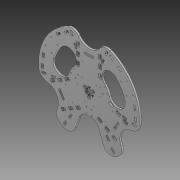
# Autodesk Inventor part: Корпус_В2_Основание
Saved by Autodesk Inventor 2022 (Build 260153000, 153)
## iProperties
Created: 2025-01-10
Part Number: Корпус_В2_Основание
Material: Типовые
Document SubType Name: Modeling
Designer: Ivan
Density: 1 g/cm^3
Appearance: Гладкий — нейтральный серый
Mass: 388.916 g
Surface Area: 1549.84 cm^2
Volume: 388.916 cm^3
Author: Ivan
Title: Корпус_В2_Основание
Autodesk Inventor part; units mm, degrees
ref_plane "YZ Plane" through (0, 0, 0) normal (1, 0, 0) x (0, 1, 0)
ref_plane "XZ Plane" through (0, 0, 0) normal (0, 1, 0) x (-1, 0, 0)
ref_plane "РабПлоскость1" through (38, -105, -570.6896) normal (0, 0, -1) x (-1, 0, 0)
sketch "Эскиз1" plane through (38, -105, -570.6896) normal (0, 0, -1) x (-1, 0, 0)
  line L0 (38, 105) -> (38, -150.1213) construction
  circle A0 centre (38, -75) radius 180
  ellipse E0 centre (38, 104.9513) end of major axis (84.5, 104.9513) minor radius 46.5 projected
  circle A1 centre (38, 104.9513) radius 46.5
  circle A2 centre (-117.8424, -164.9757) radius 46.5
  circle A3 centre (193.8424, -164.9757) radius 46.5
  point P0 (84.1166, 98.9921)
  point P1 (-8.1166, 98.9921)
  point P2 (165.6233, -201.9342)
  point P3 (211.7399, -122.0579)
  point P4 (84.1166, 98.9921)
  point P5 (84.5, 104.9513)
  point P6 (-8.1166, 98.9921)
  point P7 (-8.5, 104.9513)
  point P8 (-135.7399, -122.0579)
  point P9 (-89.6233, -201.9342)
  dimension "d0" = 180
  dimension "d6" = 360
  constraints: 3 centre point, 2 end point, 1 coincident, 1 point on line, 1 vertical, 12 other
  measures "d0" distance of point (38, -75) L0.start
extrude "Выдавливание1" add sketch "Эскиз1" along normal blind 6 contours A0 A3 A2 E0
fillet "Сопряжение1" radius 30 6 edges at (-173.7399, -227.0579, -573.6896) (-127.6233, -306.9342, -573.6896) (127.6233, -306.9342, -573.6896) (173.7399, -227.0579, -573.6896) (-46.1166, -6.0079, -573.6896) (46.1166, -6.0079, -573.6896)
sketch "Эскиз2" plane through (38, -105, -570.6896) normal (0, 0, 1) x (1, 0, 0)
  arc A0 (37.3316, 88.4783) -> (0.1581, 78.3768) centre (24.7763, 61.2319) ccw construction
  arc A1 (-76.1581, 78.3768) -> (0.1581, 78.3768) centre (-38, 104.9513) ccw construction
  arc A2 (-76.1581, 78.3768) -> (-113.3316, 88.4783) centre (-100.7763, 61.2319) ccw construction
  arc A3 (-113.3316, 88.4783) -> (-217.2421, -91.5001) centre (-38, -75) ccw construction
  arc A4 (-217.2421, -91.5001) -> (-189.9073, -118.6425) centre (-187.3685, -88.7501) ccw construction
  arc A5 (-151.7491, -184.7343) -> (-189.9073, -118.6425) centre (-193.8424, -164.9757) ccw construction
  arc A6 (-151.7491, -184.7343) -> (-141.9106, -221.9782) centre (-124.5921, -197.4818) ccw construction
  arc A7 (-141.9106, -221.9782) -> (65.9106, -221.9782) centre (-38, -75) ccw construction
  arc A8 (65.9106, -221.9782) -> (75.7491, -184.7343) centre (48.5921, -197.4818) ccw construction
  arc A9 (113.9073, -118.6425) -> (75.7491, -184.7343) centre (117.8424, -164.9757) ccw construction
  arc A10 (113.9073, -118.6425) -> (141.2421, -91.5001) centre (111.3685, -88.7501) ccw construction
  arc A11 (141.2421, -91.5001) -> (37.3316, 88.4783) centre (-38, -75) ccw construction
  circle A12 centre (-38, -75) radius 133
  circle A13 centre (-38, -75) radius 75
  line L0 (-38, -75) -> (28.5, 40.1814)
  line L1 (-38, -75) -> (95, -75)
  line L2 (-38, -75) -> (-38, -366.3532) construction
  line L3 (-38, -75) -> (208.094, 67.0824) construction
  circle A14 centre (-38, -75) radius 104 construction
  line L4 (-0.5, -10.0481) -> (28.5, 40.1814) construction
  point P0 (-38, 105)
  point P1 (37, -75)
  point P2 (-0.5, -10.0481)
  point P3 (14, 15.0666)
  dimension "d9" = 150
  dimension "d52" = 208
  dimension "d8" = 58
  dimension "d10" = 60
  dimension "d11" = 120
  constraints: 10 end point, 3 coincident, 2 point on circle, 1 centre point, 1 midpoint, 1 point on line, 1 vertical, 7 other
  measures "d10" angle of L1 L0
  measures "d11" angle of L2 L3
extrude "Выдавливание2" cut sketch "Эскиз2" against normal through all contours L1 A13 L0 A12 picked at (61.1819, -19.8946)
fillet "Сопряжение2" radius 29 4 edges at (37.5, -115.0481, -573.6896) (66.5, -64.8186, -573.6896) (75, -180, -573.6896) (133, -180, -573.6896)
mirror "Зеркальное отражение1" about plane through (0, 0, 0) normal (1, 0, 0) of "Сопряжение2", "Выдавливание2"
sketch "Эскиз3" plane through (38, -105, -570.6896) normal (0, 0, 1) x (1, 0, 0)
  circle A0 centre (-38, -75) radius 75 projected
  circle A1 centre (-38, -75) radius 133 construction
  line L0 (-38, -75) -> (25.1637, -248.5408)
  line L1 (-38, -75) -> (-101.1637, -248.5408)
  line L2 (-38, -75) -> (-38, -284.9375) construction
  circle A2 centre (-38, -75) radius 184.6782
  point P0 (-38, 105)
  point P1 (-12.3485, -145.4769)
  point P2 (-63.6515, -145.4769)
  dimension "d15" = 40
  constraints: 6 end point, 2 point on circle, 1 centre point, 1 coincident, 1 vertical, 1 other
  measures "d15" angle of L0 L1
extrude "Выдавливание3" cut sketch "Эскиз3" against normal through all contours A0 L0 A2 L1 picked at (-36.2561, -222.9049)
fillet "Сопряжение3" radius 30 4 edges at (-25.6515, -250.4769, -573.6896) (-61.5636, -349.1447, -573.6896) (25.6515, -250.4769, -573.6896) (61.5636, -349.1447, -573.6896)
sketch "Эскиз4" plane through (38, -105, -570.6896) normal (0, 0, 1) x (1, 0, 0)
  arc A0 (12.2665, -213.106) -> (56.1487, -228.4145) centre (40.4573, -202.8454) ccw construction
  arc A1 (65.9106, -221.9782) -> (75.7491, -184.7343) centre (48.5921, -197.4818) ccw construction
  arc A2 (113.9073, -118.6425) -> (75.7491, -184.7343) centre (117.8424, -164.9757) ccw construction
  arc A3 (113.9073, -118.6425) -> (141.2421, -91.5001) centre (111.3685, -88.7501) ccw construction
  arc A4 (141.2421, -91.5001) -> (37.3316, 88.4783) centre (-38, -75) ccw construction
  arc A5 (37.3316, 88.4783) -> (0.1581, 78.3768) centre (24.7763, 61.2319) ccw construction
  arc A6 (-76.1581, 78.3768) -> (0.1581, 78.3768) centre (-38, 104.9513) ccw construction
  arc A7 (-76.1581, 78.3768) -> (-113.3316, 88.4783) centre (-100.7763, 61.2319) ccw construction
  arc A8 (-113.3316, 88.4783) -> (-217.2421, -91.5001) centre (-38, -75) ccw construction
  arc A9 (-217.2421, -91.5001) -> (-189.9073, -118.6425) centre (-187.3685, -88.7501) ccw construction
  arc A10 (-151.7491, -184.7343) -> (-189.9073, -118.6425) centre (-193.8424, -164.9757) ccw construction
  arc A11 (-151.7491, -184.7343) -> (-141.9106, -221.9782) centre (-124.5921, -197.4818) ccw construction
  arc A12 (-132.1487, -228.4145) -> (-88.2665, -213.106) centre (-116.4573, -202.8454) ccw construction
  line L0 (-88.2665, -213.106) -> (-72.4151, -169.5547) construction
  arc A13 (-42.446, -149.8681) -> (-72.4151, -169.5547) centre (-44.2243, -179.8154) ccw construction
  arc A14 (-42.446, -149.8681) -> (-33.554, -149.8681) centre (-38, -75) ccw construction
  arc A15 (-3.5849, -169.5547) -> (-33.554, -149.8681) centre (-31.7757, -179.8154) ccw construction
  line L1 (-3.5849, -169.5547) -> (12.2665, -213.106) construction
  arc A16 (-133.9802, 17.0695) -> (-165.7247, -37.9135) centre (-38, -75) ccw construction
  arc A17 (-92.1242, -23.0811) -> (-110.0252, -54.0865) centre (-38, -75) ccw construction
  arc A18 (89.7247, -37.9135) -> (57.9802, 17.0695) centre (-38, -75) ccw construction
  arc A19 (34.0252, -54.0865) -> (16.1242, -23.0811) centre (-38, -75) ccw construction
  circle A20 centre (-38, -75) radius 20
  circle A21 centre (-38, -8.9997) radius 2 construction
  line L2 (-38, -8.9997) -> (-38, -75) construction
  line L3 (-38, -75) -> (8.5542, -48.1219) construction
  arc A22 (18.8589, -105.5181) -> (21.457, -107.0181) centre (19.1579, -108.0002) ccw construction
  line L4 (-38, -8.9997) -> (19.1579, -108.0002) construction
  circle A23 centre (-23.2776, -66.5) radius 5
  circle A24 centre (-38, -75) radius 17 construction
  line L5 (-28.1932, -65.5853) -> (-30.524, -66.931)
  line L6 (-24.9432, -71.2144) -> (-27.274, -72.5601)
  circle A25 centre (-38, -75) radius 11
  line L7 (-47.8068, -65.5853) -> (-45.476, -66.931)
  line L8 (-51.0568, -71.2144) -> (-48.726, -72.5601)
  circle A26 centre (-52.7224, -66.5) radius 5
  line L9 (-41.25, -88.2003) -> (-41.25, -85.5089)
  line L10 (-34.75, -88.2003) -> (-34.75, -85.5089)
  circle A27 centre (-38, -92) radius 5
  line L11 (-43, -59) -> (-33, -59)
  line L12 (-33, -59) -> (-33, -61)
  line L13 (-33, -61) -> (-43, -61)
  line L14 (-43, -61) -> (-43, -59)
  line L15 (-43, -59) -> (-33, -61) construction
  line L16 (-33, -59) -> (-43, -61) construction
  line L17 (-37, -61) -> (-37, -64.0455)
  line L18 (-39, -61) -> (-39, -64.0455)
  line L19 (-49.6244, -82.866) -> (-46.9868, -81.3433)
  line L20 (-50.6244, -81.134) -> (-47.9868, -79.6112)
  line L21 (-54.3564, -78.6699) -> (-52.6244, -77.6699)
  line L22 (-47.6244, -86.3301) -> (-49.3564, -87.3301)
  line L23 (-52.6244, -77.6699) -> (-47.6244, -86.3301)
  line L24 (-49.3564, -87.3301) -> (-54.3564, -78.6699)
  line L25 (-49.3564, -87.3301) -> (-52.6244, -77.6699) construction
  line L26 (-54.3564, -78.6699) -> (-47.6244, -86.3301) construction
  line L27 (-25.3756, -81.134) -> (-28.0132, -79.6112)
  line L28 (-26.3756, -82.866) -> (-29.0132, -81.3433)
  line L29 (-26.6436, -87.3301) -> (-28.3756, -86.3301)
  line L30 (-23.3756, -77.6699) -> (-21.6436, -78.6699)
  line L31 (-28.3756, -86.3301) -> (-23.3756, -77.6699)
  line L32 (-21.6436, -78.6699) -> (-26.6436, -87.3301)
  line L33 (-21.6436, -78.6699) -> (-28.3756, -86.3301) construction
  line L34 (-26.6436, -87.3301) -> (-23.3756, -77.6699) construction
  arc A28 (-165.7247, -37.9135) -> (-110.0252, -54.0865) centre (-137.8749, -46) ccw projected
  arc A29 (-92.1242, -23.0811) -> (-133.9802, 17.0695) centre (-113.0522, -3.0058) ccw projected
  arc A30 (57.9802, 17.0695) -> (16.1242, -23.0811) centre (37.0522, -3.0058) ccw projected
  arc A31 (34.0252, -54.0865) -> (89.7247, -37.9135) centre (61.8749, -46) ccw projected
  arc A32 (56.1487, -228.4145) -> (65.9106, -221.9782) centre (-38, -75) ccw projected
  arc A33 (-141.9106, -221.9782) -> (-132.1487, -228.4145) centre (-38, -75) ccw projected
  point P0 (-38, 105)
  point P1 (-38, -60)
  point P2 (-50.9904, -82.5)
  point P3 (-25.0096, -82.5)
  point P4 (-28.0132, -79.6112)
  point P5 (-45.476, -66.931)
  point P6 (-47.9868, -79.6112)
  point P7 (-46.9868, -81.3433)
  point P8 (-41.25, -85.5089)
  point P9 (-29.0132, -81.3433)
  dimension "d21" = 34
  dimension "d19" = 40
  dimension "d20" = 10
  dimension "d22" = 6.5
  dimension "d23" = 22
  dimension "d26" = 360
  dimension "d28" = 10
  dimension "d29" = 2
  dimension "d30" = 2
  dimension "d31" = 15
  dimension "d34" = 360
  constraints: 66 end point, 10 point on circle, 8 point on line, 6 midpoint, 5 centre point, 4 parallel, 3 coincident, 2 perpendicular, 2 vertical, 1 horizontal, 82 other
  measures "d19" diameter of A20
  measures "d20" diameter of A23
  measures "d22" distance between parallel lines of L5 L6
  measures "d23" diameter of A25
  measures "d28" distance of L12.end L13.end
  measures "d29" distance of L11.end L12.end
  measures "d30" distance between parallel lines of L18 L17
  measures "d31" distance of A16.centre point (-38, -60)
extrude "Выдавливание4" cut sketch "Эскиз4" against normal through all contours A23 A20 | A20 A23 | A27 A20 | A20 A27 | L6 A25 L5 A23 | A26 A20 | A20 A26 | A25 | L9 A25 L10 A27 | L7 A25 L8 A26 | A25 L18 L13 L17 | L27 L31 L28 A25 | L19 L23 L20 A25 | L13 L14 L11 L12 | L31 L30 L32 L29 | L23 L22 L24 L21
fillet "Сопряжение4" radius 1 24 edges at (9.9868, -184.6112, -573.6896) (8.9868, -186.3433, -573.6896) (10.726, -177.5601, -573.6896) (7.476, -171.931, -573.6896) (1, -169.0455, -573.6896) (-1, -169.0455, -573.6896) (-7.476, -171.931, -573.6896) (-10.726, -177.5601, -573.6896) (-8.9868, -186.3433, -573.6896) (-9.9868, -184.6112, -573.6896) (-3.25, -190.5089, -573.6896) (3.25, -190.5089, -573.6896) (11.6244, -187.866, -573.6896) (12.6244, -186.134, -573.6896) (-11.6244, -187.866, -573.6896) (-12.6244, -186.134, -573.6896) (1, -166, -573.6896) (-1, -166, -573.6896) (-9.8068, -170.5853, -573.6896) (-13.0568, -176.2144, -573.6896) (9.8068, -170.5853, -573.6896) (13.0568, -176.2144, -573.6896) (3.25, -193.2003, -573.6896) (-3.25, -193.2003, -573.6896)
sketch "Эскиз5" plane through (38, -105, -576.6896) normal (0, 0, -1) x (-1, 0, 0)
  arc A0 (217.2421, -91.5001) -> (113.3316, 88.4783) centre (38, -75) ccw construction
  arc A1 (217.2421, -91.5001) -> (113.3316, 88.4783) centre (38, -75) ccw construction
  arc A2 (36.1667, -64.1539) -> (31.0391, -66.4826) centre (38, -75) ccw construction
  arc A3 (88.2665, -213.106) -> (132.1487, -228.4145) centre (116.4573, -202.8454) ccw construction
  line L0 (38, -75) -> (116.4573, -202.8454) construction
  line L1 (124.3613, -221.4606) -> (98.2089, -178.8455)
  line L2 (98.2089, -178.8455) -> (103.3227, -175.7072)
  line L3 (103.3227, -175.7072) -> (129.4751, -218.3224)
  line L4 (129.4751, -218.3224) -> (124.3613, -221.4606)
  line L5 (124.3613, -221.4606) -> (103.3227, -175.7072) construction
  line L6 (98.2089, -178.8455) -> (129.4751, -218.3224) construction
  line L7 (106.0546, -191.63) -> (111.1685, -188.4918)
  line L8 (121.6294, -205.5378) -> (116.5156, -208.6761)
  line L9 (113.842, -198.5839) -> (116.3989, -197.0148) construction
  circle A4 centre (38, -75) radius 145 construction
  line L10 (38, -75) -> (215.7726, -98.4042) construction
  arc A5 (189.9073, -118.6425) -> (217.2421, -91.5001) centre (187.3685, -88.7501) ccw construction
  line L11 (38, -75) -> (106.6177, 90.6577) construction
  arc A6 (113.3316, 88.4783) -> (76.1581, 78.3768) centre (100.7763, 61.2319) ccw construction
  line L12 (38, -75) -> (193.8846, 15) construction
  arc A7 (217.2421, -91.5001) -> (113.3316, 88.4783) centre (38, -75) ccw construction
  line L13 (206.154, -100.1638) -> (156.5818, -93.6375)
  line L14 (156.5818, -93.6375) -> (157.365, -87.6888)
  line L15 (157.365, -87.6888) -> (206.9372, -94.2151)
  line L16 (206.9372, -94.2151) -> (206.154, -100.1638)
  line L17 (206.154, -100.1638) -> (157.365, -87.6888) construction
  line L18 (156.5818, -93.6375) -> (206.9372, -94.2151) construction
  line L19 (171.4535, -95.5954) -> (172.2366, -89.6467)
  line L20 (192.0655, -92.2572) -> (191.2824, -98.2059)
  line L21 (181.7595, -93.9263) -> (182.1511, -90.952) construction
  line L22 (81.1504, 37.0136) -> (100.2845, 83.2076)
  line L23 (100.2845, 83.2076) -> (105.8278, 80.9115)
  line L24 (105.8278, 80.9115) -> (86.6937, 34.7175)
  line L25 (86.6937, 34.7175) -> (81.1504, 37.0136)
  line L26 (81.1504, 37.0136) -> (105.8278, 80.9115) construction
  line L27 (100.2845, 83.2076) -> (86.6937, 34.7175) construction
  line L28 (94.5443, 69.3494) -> (100.0876, 67.0533)
  line L29 (92.4339, 48.5757) -> (86.8906, 50.8718)
  line L30 (93.4891, 58.9625) -> (96.2607, 57.8145) construction
  line L31 (203.1818, -35.453) -> (207.5396, -85.2627)
  line L32 (207.5396, -85.2627) -> (201.5624, -85.7856)
  line L33 (201.5624, -85.7856) -> (197.2046, -35.9759)
  line L34 (197.2046, -35.9759) -> (203.1818, -35.453)
  line L35 (203.1818, -35.453) -> (201.5624, -85.7856) construction
  line L36 (207.5396, -85.2627) -> (197.2046, -35.9759) construction
  line L37 (206.2323, -70.3198) -> (200.2551, -70.8427)
  line L38 (204.4892, -50.3959) -> (198.512, -50.9188)
  line L39 (202.3721, -60.6193) -> (199.3835, -60.8808) construction
  circle A8 centre (38, -75) radius 165 construction
  line L40 (202.3721, -60.6193) -> (204.551, -85.5242) construction
  line L41 (38, -75) -> (38, 24.0008) construction
  line L42 (154.8396, 48.2781) -> (113.882, 76.957)
  line L43 (113.882, 76.957) -> (110.4406, 72.042)
  line L44 (110.4406, 72.042) -> (151.3982, 43.3632)
  line L45 (151.3982, 43.3632) -> (154.8396, 48.2781)
  line L46 (154.8396, 48.2781) -> (110.4406, 72.042) construction
  line L47 (113.882, 76.957) -> (151.3982, 43.3632) construction
  line L48 (126.1693, 68.3533) -> (122.7279, 63.4384)
  line L49 (142.5524, 56.8818) -> (139.1109, 51.9669)
  line L50 (132.6401, 60.1601) -> (130.9194, 57.7026) construction
  line L51 (132.6401, 60.1601) -> (112.1613, 74.4995) construction
  point P0 (38, 105)
  point P1 (132.127, -206.5631)
  point P2 (156.9734, -90.6631)
  point P3 (93.4891, 58.9625)
  point P4 (103.0562, 82.0595)
  dimension "d60" = 330
  dimension "d39" = 6
  dimension "d40" = 50
  dimension "d41" = 15
  dimension "d42" = 290
  dimension "d45" = 75
  dimension "d46" = 6
  dimension "d47" = 50
  dimension "d48" = 15
  dimension "d49" = 6
  dimension "d50" = 50
  dimension "d51" = 15
  dimension "d58" = 15
  dimension "d59" = 15
  dimension "d61" = 85
  constraints: 104 end point, 25 point on line, 20 midpoint, 13 perpendicular, 12 symmetric about line, 8 parallel, 7 point on circle, 2 coincident, 2 equal length, 1 centre point, 1 vertical, 8 other
  measures "d39" distance of L3.end L1.start
  measures "d40" distance of L2.end L3.end
  measures "d41" distance between parallel lines of L4 L8
  measures "d42" diameter of A4
  measures "d45" angle of L11 L10
  measures "d46" distance of L15.end L16.end
  measures "d47" distance of L14.end L15.end
  measures "d48" distance between parallel lines of L16 L20
  measures "d49" distance of L24.end L25.end
  measures "d50" distance of L23.end L24.end
  measures "d51" distance between parallel lines of L25 L29
  measures "d58" distance between parallel lines of L34 L38
  measures "d59" distance between parallel lines of L32 L37
  measures "d61" angle of L39 L41
extrude "Выдавливание5" cut sketch "Эскиз5" against normal through all contours L1 L8 L3 L4 | L1 L2 L3 L7 | L13 L20 L15 L16 | L13 L14 L15 L19 | L22 L29 L24 L25 | L22 L23 L24 L28 | L31 L38 L33 L34 | L31 L32 L33 L37 | L45 L44 L49 L42 | L48 L44 L43 L42
mirror "Зеркальное отражение2" about plane through (0, 0, 0) normal (1, 0, 0) of "Выдавливание5"
sketch "Эскиз6" plane through (38, -105, -570.6896) normal (0, 0, 1) x (1, 0, 0)
  line L0 (100.9134, -104.3949) -> (87.923, -96.8949) projected
  line L1 (99.4134, -106.993) -> (100.9134, -104.3949) projected
  line L2 (86.423, -99.493) -> (87.923, -96.8949) projected
  line L3 (83.423, -104.6891) -> (84.923, -102.091) projected
  line L4 (84.923, -102.091) -> (86.423, -99.493) projected
  line L5 (97.9134, -109.591) -> (99.4134, -106.993) projected
  line L6 (96.4134, -112.1891) -> (97.9134, -109.591) projected
  line L7 (96.4134, -112.1891) -> (83.423, -104.6891) projected
  line L8 (73.4327, -91.993) -> (74.9327, -89.3949) projected
  line L9 (74.9327, -89.3949) -> (61.9423, -81.8949) projected
  line L10 (71.9327, -94.591) -> (73.4327, -91.993) projected
  line L11 (70.4327, -97.1891) -> (71.9327, -94.591) projected
  line L12 (70.4327, -97.1891) -> (57.4423, -89.6891) projected
  line L13 (57.4423, -89.6891) -> (58.9423, -87.091) projected
  line L14 (58.9423, -87.091) -> (60.4423, -84.493) projected
  line L15 (60.4423, -84.493) -> (61.9423, -81.8949) projected
  line L16 (49.7628, -142.9904) -> (64.7628, -117.0096) projected
  line L17 (64.7628, -117.0096) -> (69.9589, -120.0096) projected
  line L18 (54.9589, -145.9904) -> (69.9589, -120.0096) projected
  line L19 (49.7628, -142.9904) -> (54.9589, -145.9904) projected
  line L20 (48.423, -165.3109) -> (61.4134, -172.8109) projected
  line L21 (61.4134, -172.8109) -> (59.9134, -175.409) projected
  line L22 (46.923, -167.909) -> (59.9134, -175.409) projected
  line L23 (48.423, -165.3109) -> (46.923, -167.909) projected
  line L24 (46.923, -167.909) -> (59.9134, -175.409) projected
  line L25 (59.9134, -175.409) -> (58.4134, -178.007) projected
  line L26 (45.423, -170.507) -> (58.4134, -178.007) projected
  line L27 (46.923, -167.909) -> (45.423, -170.507) projected
  line L28 (45.423, -170.507) -> (58.4134, -178.007) projected
  line L29 (58.4134, -178.007) -> (56.9134, -180.6051) projected
  line L30 (43.923, -173.1051) -> (56.9134, -180.6051) projected
  line L31 (45.423, -170.507) -> (43.923, -173.1051) projected
  line L32 (22.4423, -150.3109) -> (35.4327, -157.8109) projected
  line L33 (35.4327, -157.8109) -> (33.9327, -160.409) projected
  line L34 (20.9423, -152.909) -> (33.9327, -160.409) projected
  line L35 (22.4423, -150.3109) -> (20.9423, -152.909) projected
  line L36 (20.9423, -152.909) -> (33.9327, -160.409) projected
  line L37 (33.9327, -160.409) -> (32.4327, -163.007) projected
  line L38 (19.4423, -155.507) -> (32.4327, -163.007) projected
  line L39 (20.9423, -152.909) -> (19.4423, -155.507) projected
  line L40 (19.4423, -155.507) -> (32.4327, -163.007) projected
  line L41 (32.4327, -163.007) -> (30.9327, -165.6051) projected
  line L42 (17.9423, -158.1051) -> (30.9327, -165.6051) projected
  line L43 (19.4423, -155.507) -> (17.9423, -158.1051) projected
  line L44 (99.4134, -106.993) -> (86.423, -99.493) projected
  line L45 (86.423, -99.493) -> (87.923, -96.8949) projected
  line L46 (100.9134, -104.3949) -> (87.923, -96.8949) projected
  line L47 (99.4134, -106.993) -> (100.9134, -104.3949) projected
  line L48 (97.9134, -109.591) -> (84.923, -102.091) projected
  line L49 (84.923, -102.091) -> (86.423, -99.493) projected
  line L50 (99.4134, -106.993) -> (86.423, -99.493) projected
  line L51 (97.9134, -109.591) -> (99.4134, -106.993) projected
  line L52 (96.4134, -112.1891) -> (83.423, -104.6891) projected
  line L53 (83.423, -104.6891) -> (84.923, -102.091) projected
  line L54 (97.9134, -109.591) -> (84.923, -102.091) projected
  line L55 (96.4134, -112.1891) -> (97.9134, -109.591) projected
  line L56 (47.4519, -76.993) -> (34.4615, -69.493) projected
  line L57 (34.4615, -69.493) -> (35.9615, -66.8949) projected
  line L58 (48.9519, -74.3949) -> (35.9615, -66.8949) projected
  line L59 (47.4519, -76.993) -> (48.9519, -74.3949) projected
  line L60 (45.9519, -79.591) -> (32.9615, -72.091) projected
  line L61 (32.9615, -72.091) -> (34.4615, -69.493) projected
  line L62 (47.4519, -76.993) -> (34.4615, -69.493) projected
  line L63 (45.9519, -79.591) -> (47.4519, -76.993) projected
  line L64 (44.4519, -82.1891) -> (31.4615, -74.6891) projected
  line L65 (31.4615, -74.6891) -> (32.9615, -72.091) projected
  line L66 (45.9519, -79.591) -> (32.9615, -72.091) projected
  line L67 (44.4519, -82.1891) -> (45.9519, -79.591) projected
  line L68 (73.4327, -91.993) -> (60.4423, -84.493) projected
  line L69 (60.4423, -84.493) -> (61.9423, -81.8949) projected
  line L70 (74.9327, -89.3949) -> (61.9423, -81.8949) projected
  line L71 (73.4327, -91.993) -> (74.9327, -89.3949) projected
  line L72 (70.4327, -97.1891) -> (57.4423, -89.6891) projected
  line L73 (57.4423, -89.6891) -> (58.9423, -87.091) projected
  line L74 (71.9327, -94.591) -> (58.9423, -87.091) projected
  line L75 (70.4327, -97.1891) -> (71.9327, -94.591) projected
  line L76 (71.9327, -94.591) -> (58.9423, -87.091) projected
  line L77 (58.9423, -87.091) -> (60.4423, -84.493) projected
  line L78 (73.4327, -91.993) -> (60.4423, -84.493) projected
  line L79 (71.9327, -94.591) -> (73.4327, -91.993) projected
  line L80 (-3.5385, -135.3109) -> (9.4519, -142.8109) projected
  line L81 (9.4519, -142.8109) -> (7.9519, -145.409) projected
  line L82 (-5.0385, -137.909) -> (7.9519, -145.409) projected
  line L83 (-3.5385, -135.3109) -> (-5.0385, -137.909) projected
  line L84 (-5.0385, -137.909) -> (7.9519, -145.409) projected
  line L85 (7.9519, -145.409) -> (6.4519, -148.007) projected
  line L86 (-6.5385, -140.507) -> (6.4519, -148.007) projected
  line L87 (-5.0385, -137.909) -> (-6.5385, -140.507) projected
  line L88 (-6.5385, -140.507) -> (6.4519, -148.007) projected
  line L89 (6.4519, -148.007) -> (4.9519, -150.6051) projected
  line L90 (-8.0385, -143.1051) -> (4.9519, -150.6051) projected
  line L91 (-6.5385, -140.507) -> (-8.0385, -143.1051) projected
  point P0 (-38, 105)
  constraints: 1 other
extrude "Выдавливание6" cut sketch "Эскиз6" against normal through all
pattern_circular "Круговой массив1" count 3 over 360 about axis through (0, -180, -570.6896) along (0, 0, -1) of "Выдавливание6"
sketch "Эскиз7" plane through (38, -105, -570.6896) normal (0, 0, 1) x (1, 0, 0)
  arc A0 (-113.3316, 88.4783) -> (-217.2421, -91.5001) centre (-38, -75) ccw projected
  line L0 (162, -225) -> (-238, -225)
  line L1 (-238, -225) -> (-238, 75)
  line L2 (-238, 75) -> (162, 75)
  line L3 (162, 75) -> (162, -225)
  line L4 (162, -225) -> (-238, 75) construction
  line L5 (-238, -225) -> (162, 75) construction
  line L6 (220.7514, -288.1285) -> (-335.7827, -288.1285)
  line L7 (-335.7827, -288.1285) -> (-335.7827, 148.337)
  line L8 (-335.7827, 148.337) -> (220.7514, 148.337)
  line L9 (220.7514, 148.337) -> (220.7514, -288.1285)
  point P0 (-38, 105)
  dimension "d64" = 300
  dimension "d65" = 400
  constraints: 20 end point, 4 parallel, 2 horizontal, 2 midpoint, 2 perpendicular
  measures "d64" distance of L0.end L1.end
  measures "d65" distance of L0.start L0.end
extrude "Выдавливание7" [suppressed]
sketch "Эскиз8" plane through (38, -105, -570.6896) normal (0, 0, 1) x (1, 0, 0)
  circle A0 centre (-13, -42.5) radius 3 construction
  circle A1 centre (-13, 7.5) radius 3 construction
  circle A2 centre (-63, -42.5) radius 3 construction
  circle A3 centre (-63, 7.5) radius 3 construction
  point P0 (-38, 105)
  constraints: 4 coincident
hole "Отверстие1" at (25, -147.5, -570.6896) at (25, -97.5, -570.6896) at (-25, -147.5, -570.6896) at (-25, -97.5, -570.6896) direction (0, 0, -1) diameter 1.5 end through all
pattern_circular "Круговой массив2" count 3 over 360 about axis through (0, -180, -570.6896) along (0, 0, -1) of "Отверстие1"
sketch "Эскиз9" plane through (38, -105, -570.6896) normal (0, 0, 1) x (1, 0, 0)
  arc A0 (56.1487, -228.4145) -> (65.9106, -221.9782) centre (-38, -75) ccw construction
  line L0 (-38, -75) -> (-38, -194.1828) construction
  line L1 (-29, -144) -> (-47, -144) construction
  line L2 (-47, -144) -> (-47, -126) construction
  line L3 (-47, -126) -> (-29, -126) construction
  line L4 (-29, -126) -> (-29, -144) construction
  line L5 (-29, -144) -> (-47, -126) construction
  line L6 (-47, -144) -> (-29, -126) construction
  circle A1 centre (-38, -75) radius 60 construction
  point P0 (-38, 105)
  point P1 (-217.2421, -91.5001)
  point P2 (-137.4987, 75)
  point P3 (-38, -135)
  point P4 (10.6673, -57.2942)
  point P5 (1.6673, -41.7058)
  point P6 (17.2558, -32.7058)
  point P7 (26.2558, -48.2942)
  point P8 (-77.6673, -41.7058)
  point P9 (-86.6673, -57.2942)
  point P10 (-102.2558, -48.2942)
  point P11 (-93.2558, -32.7058)
  dimension "d78" = 60
  dimension "d79" = 18
  dimension "d89" = 360
  constraints: 14 end point, 5 coincident, 2 midpoint, 2 parallel, 2 perpendicular, 1 horizontal, 1 point on line, 1 vertical, 1 vertical alignment, 15 other
  measures "d78" distance of L0.start point (-38, -135)
  measures "d79" distance of L2.end L3.end
hole "Отверстие2" at (-9, -231, -570.6896) at (9, -231, -570.6896) at (9, -249, -570.6896) at (-9, -249, -570.6896) at (-48.6673, -162.2942, -570.6896) at (-39.6673, -146.7058, -570.6896) at (-55.2558, -137.7058, -570.6896) at (-64.2558, -153.2942, -570.6896) at (64.2558, -153.2942, -570.6896) at (55.2558, -137.7058, -570.6896) at (39.6673, -146.7058, -570.6896) at (48.6673, -162.2942, -570.6896) direction (0, 0, -1) diameter 3.2 end through all clearance for "болты с шестигранной головкой / гайка ГОСТ 12876-67" size "M3" standard "ГОСТ"
sketch "Эскиз10" plane through (38, -105, -570.6896) normal (0, 0, 1) x (1, 0, 0)
  arc A0 (56.1487, -228.4145) -> (65.9106, -221.9782) centre (-38, -75) ccw construction
  arc A1 (-133.9802, 17.0695) -> (-165.7247, -37.9135) centre (-38, -75) ccw construction
  line L0 (-38, -75) -> (-288.4711, 69.6096) construction
  line L1 (-151.4086, 13.5705) -> (-171.4086, -21.0705) construction
  line L2 (-171.4086, -21.0705) -> (-193.0593, -8.5705) construction
  line L3 (-193.0593, -8.5705) -> (-173.0593, 26.0705) construction
  line L4 (-173.0593, 26.0705) -> (-151.4086, 13.5705) construction
  line L5 (-151.4086, 13.5705) -> (-193.0593, -8.5705) construction
  line L6 (-171.4086, -21.0705) -> (-173.0593, 26.0705) construction
  point P0 (-38, 105)
  point P1 (-217.2421, -91.5001)
  point P2 (-137.4987, 75)
  point P3 (-153.1814, -8.5)
  point P4 (-172.2339, 2.5)
  dimension "d91" = 40
  dimension "d92" = 25
  dimension "d93" = 155
  constraints: 14 end point, 4 coincident, 2 midpoint, 2 parallel, 2 perpendicular, 2 point on line, 1 point on circle
  measures "d91" distance of L2.end L3.end
  measures "d92" distance of L1.end L2.end
  measures "d93" distance of A0.centre point (-172.234, 2.5)
hole "Отверстие3" at (-133.4086, -126.0705, -570.6896) at (-155.0593, -113.5705, -570.6896) at (-113.4086, -91.4295, -570.6896) at (-135.0593, -78.9295, -570.6896) direction (0, 0, -1) diameter 3.2 end through all clearance for "болты с шестигранной головкой / гайка ГОСТ 12876-67" size "M3" standard "ГОСТ"
mirror "Зеркальное отражение3" about plane through (0, 0, 0) normal (1, 0, 0) of "Отверстие3"
equation "\"d22\" = 0.65 * d20"
